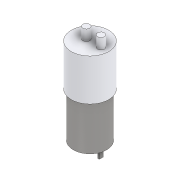
# Autodesk Inventor part: Pumpe_Dummy
Saved by Autodesk Inventor 2020 (Build 240168000, 168)
## iProperties
Created: 2020-08-23
Part Number: Pumpe_Dummy
Material: Generisch
Document SubType Name: Modeling
Designer: uhlma
Density: 1 g/cm^3
Appearance: Galvanisiert
Author: uhlma
Autodesk Inventor part; units mm, degrees
ref_plane "YZ Plane" through (0, 0, 0) normal (1, 0, 0) x (0, 1, 0)
ref_plane "XZ Plane" through (0, 0, 0) normal (0, 1, 0) x (-1, 0, 0)
ref_plane "XY Plane" through (0, 0, 0) normal (0, 0, 1) x (1, 0, 0)
sketch "Skizze1" plane through (0, 0, 0) normal (0, 0, 1) x (1, 0, 0)
  line L0 (0, 0) -> (0, 47.086)
  line L1 (0, 43.9) -> (-9.5, 43.9)
  line L2 (-9.5, 43.9) -> (-9.5, 22.7)
  line L3 (-9.5, 22.7) -> (-8.5, 22.7)
  line L4 (-8.5, 22.7) -> (-8.5, 0)
  line L5 (-8.5, 0) -> (0, 0)
  dimension "d0" = 19
  dimension "d1" = 17
  dimension "d2" = 43.9
  dimension "d3" = 21.2
  constraints: 12 end point, 5 perpendicular, 1 point on line, 1 vertical
  measures "d0" diameter of L2 L0
  measures "d1" diameter of L4 L0
  measures "d2" distance between parallel lines of L5 L1
  measures "d3" distance from line of L1 L3.end
revolve "Umdrehung1" add sketch "Skizze1" angle 360 about axis through (0, 0, 0) along (0, 1, 0)
sketch "Skizze2" plane through (0, 0, 0) normal (0, -1, 0) x (1, 0, 0)
  line L0 (5.7629, 1.0144) -> (5, 1.0144)
  line L1 (5, 1.0144) -> (5, -1.0144)
  line L2 (5, -1.0144) -> (5.7629, -1.0144)
  line L3 (5.7629, -1.0144) -> (5.7629, 1.0144)
  point P0 (0, 0)
  point P1 (5.7629, 0)
  dimension "d5" = 5
  constraints: 8 end point, 2 parallel, 1 horizontal, 1 horizontal alignment, 1 midpoint, 1 perpendicular
  measures "d5" distance from line of point (0, 0) L1
extrude "Extrusion1" add sketch "Skizze2" along normal blind 5
mirror "Spiegeln1" about plane through (0, 0, 0) normal (1, 0, 0) of "Extrusion1"
sketch "Skizze3" plane through (0, 43.9, 0) normal (0, 1, 0) x (1, 0, 0)
  circle A0 centre (-1.8885, 0) radius 1.75
  circle A1 centre (5.6115, 0) radius 1.75
  point P0 (0, 0)
  dimension "d8" = 7.5
  dimension "d9" = 3.5
  constraints: 2 centre point, 2 horizontal alignment, 1 equal radius
  measures "d8" distance of A1.centre A0.centre
  measures "d9" diameter of A0
extrude "Extrusion2" add sketch "Skizze3" along normal blind 5.5
